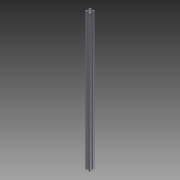
# Autodesk Inventor part: Alu-Profil Nut 8 30x30 870
Saved by Autodesk Inventor 2012 SP1 (Build 160190100, 190)
## iProperties
Created: 2013-01-29
Part Number: Alu-Profil Nut 8 30x30 870
Material: Default
Document SubType Name: Modeling
Designer: vogel
Density: 1 g/cm^3
Author: vogel
Autodesk Inventor part; units mm, degrees
ref_plane "YZ Plane" through (0, 0, 0) normal (1, 0, 0) x (0, 1, 0)
ref_plane "XZ Plane" through (0, 0, 0) normal (0, 1, 0) x (-1, 0, 0)
ref_plane "XY Plane" through (0, 0, 0) normal (0, 0, 1) x (1, 0, 0)
sketch "Skizze1" plane through (0, 0, 0) normal (0, 0, 1) x (1, 0, 0)
  line L0 (-13, 15) -> (13, 15)
  line L1 (15, 13) -> (15, -13)
  line L2 (13, -15) -> (-13, -15)
  line L3 (-15, -13) -> (-15, 13)
  circle A0 centre (0, 0) radius 3.5
  line L4 (-21.5799, 0) -> (21.5799, 0) projected
  line L5 (0, -21.5799) -> (0, 21.5799) projected
  arc A1 (15, 13) -> (13, 15) centre (13, 13) ccw
  arc A2 (-13, 15) -> (-15, 13) centre (-13, 13) ccw
  arc A3 (-15, -13) -> (-13, -15) centre (-13, -13) ccw
  arc A4 (13, -15) -> (15, -13) centre (13, -13) ccw
  point P0 (-15, 15)
  point P1 (15, 15)
  point P2 (-15, -15)
  dimension "d0" = 30
  dimension "d1" = 30
  dimension "d2" = 7
  dimension "d3" = 2
  constraints: 8 end point, 8 point on circle, 8 tangent, 6 point on line, 5 centre point, 3 equal radius, 2 parallel, 1 coincident, 1 horizontal, 1 perpendicular, 2 other
  measures "d0" distance of point (-15, -15) point (-15, 15)
  measures "d1" distance of point (-15, 15) point (15, 15)
  measures "d2" diameter of A0
  measures "d3" radius of A1
extrude "Extrusion1" add sketch "Skizze1" along normal blind 870 contours L0 L5 A0 L4 L3 A2 | L0 A1 L1 L4 A0 L5 | L4 A0 L5 L2 A3 L3 | L4 L1 A4 L2 L5 A0
sketch "Skizze2" plane through (0, 0, 0) normal (0, 0, -1) x (-1, 0, 0)
  line L0 (13, -15) -> (-13, -15) projected
  line L1 (21, 0) -> (-21, 0) projected
  line L2 (0, -21) -> (0, 21) projected
  line L3 (-6, -15) -> (-6, -14.5)
  line L4 (-6, -14.5) -> (-4, -14.5)
  line L5 (-4, -14.5) -> (-4, -12.5)
  line L6 (-4, -12.5) -> (-7.5, -12.5)
  line L7 (-7.5, -12.5) -> (-7.5, -9)
  line L8 (-7.5, -9) -> (-4.4, -5.9)
  line L9 (-4.4, -5.9) -> (4.4, -5.9)
  line L10 (4.4, -5.9) -> (7.5, -9)
  line L11 (7.5, -9) -> (7.5, -12.5)
  line L12 (7.5, -12.5) -> (4, -12.5)
  line L13 (4, -12.5) -> (4, -14.5)
  line L14 (4, -14.5) -> (6, -14.5)
  line L15 (6, -14.5) -> (6, -15)
  dimension "d6" = 8
  dimension "d7" = 15
  dimension "d8" = 12
  dimension "d9" = 0.5
  dimension "d10" = 9.1
  dimension "d11" = 135
  dimension "d12" = 2.5
  dimension "d13" = 3.5
  constraints: 26 end point, 8 parallel, 3 collinear, 2 perpendicular, 2 point on line, 4 other
  measures "d6" distance between parallel lines of L5 L13
  measures "d7" distance between parallel lines of L11 L7
  measures "d8" distance between parallel lines of L3 L15
  measures "d9" distance between parallel lines of L14 L0
  measures "d10" distance between parallel lines of L9 L0
  measures "d11" angle of L9 L10
  measures "d12" distance between parallel lines of L0 L12
  measures "d13" distance of L10.end L11.end
extrude "Extrusion2" cut sketch "Skizze2" against normal through all
pattern_circular "Runde Anordnung1" count 4 over 360 about axis through (0, 0, 0) along (0, 0, 1) of "Extrusion2"
sketch "Skizze3" plane through (0, 0, 0) normal (0, 0, -1) x (-1, 0, 0)
  circle A0 centre (0, 0) radius 3.5 projected
  line L0 (21, 0) -> (-21, 0) projected
  line L1 (0, -21) -> (0, 21) projected
  line L2 (-1, 4.3875) -> (-1, 3.3541)
  line L3 (1, 4.3875) -> (1, 3.3541)
  arc A1 (1, 4.3875) -> (-1, 4.3875) centre (0, 0) ccw
  dimension "d20" = 2
  dimension "d21" = 2
  dimension "d22" = 4.5
  constraints: 4 end point, 4 point on circle, 1 centre point, 1 coincident, 1 other
  measures "d20" distance of L3.end L2.end
  measures "d21" distance of L3.start L2.start
  measures "d22" radius of A1
extrude "Extrusion3" cut sketch "Skizze3" against normal through all contours A0 L1 A1 L3 | A0 L2 A1 L1
pattern_circular "Runde Anordnung2" count 6 over 360 about axis through (0, 0, 0) along (0, 0, 1) of "Extrusion3"
